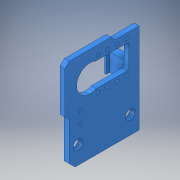
# Autodesk Inventor part: КВ33.044.002 - Деражатель мотора
Saved by Autodesk Inventor 2019 (Build 230136000, 136)
## iProperties
Created: 2019-07-16
Part Number: КВ33.044.002 - Деражатель мотора
Material: Пластик АБС
Document SubType Name: Modeling
Designer: user
Density: 1.06 g/cm^3
Appearance: Голубой
Mass: 13.0069 g
Surface Area: 83.1984 cm^2
Volume: 12.2706 cm^3
Author: user
Autodesk Inventor part; units mm, degrees
ref_plane "YZ Plane" through (0, 0, 0) normal (1, 0, 0) x (0, 1, 0)
ref_plane "XZ Plane" through (0, 0, 0) normal (0, 1, 0) x (-1, 0, 0)
ref_plane "XY Plane" through (0, 0, 0) normal (0, 0, 1) x (1, 0, 0)
sketch "Эскиз1" plane through (0, 0, 0) normal (1, 0, 0) x (0, 1, 0)
  line L0 (-17.5, 21) -> (-21, 17.5)
  line L1 (-21, 17.5) -> (-21, -17.5)
  line L2 (-21, -17.5) -> (-17.5, -21)
  line L3 (-17.5, -21) -> (17.5, -21)
  line L4 (17.5, -21) -> (21, -17.5)
  line L5 (21, -17.5) -> (21, 17.5)
  line L6 (21, 17.5) -> (17.5, 21)
  line L7 (17.5, 21) -> (-17.5, 21)
  circle A0 centre (0, 0) radius 10.75
  circle A1 centre (-15.5, -15.5) radius 1.25
  circle A2 centre (15.5, -15.5) radius 1.25
  circle A3 centre (15.5, 15.5) radius 1.25
  circle A4 centre (-15.5, 15.5) radius 1.25
  line L8 (-21, 17.5) -> (-58, 17.5)
  line L9 (-58, 17.5) -> (-58, -17.5)
  line L10 (-58, -17.5) -> (-21, -17.5)
  line L11 (-21, -17.5) -> (-21, 17.5)
  line L12 (-58, 0) -> (-43, 0)
  line L13 (-43, 0) -> (-43, 10)
  circle A5 centre (-43, 10) radius 4
  circle A6 centre (-43, -33.5) radius 4
  line L14 (-58, -17.5) -> (-17.5, -17.5)
  line L15 (-17.5, -17.5) -> (-17.5, -41)
  line L16 (-17.5, -41) -> (-58, -41)
  line L17 (-58, -41) -> (-58, -17.5)
  dimension "d0" = 37
  dimension "d1" = 15
  dimension "d2" = 10
  dimension "d4" = 8
  dimension "d5" = 8
  dimension "d12" = 21.5
  dimension "d115" = 40.5
  dimension "d116" = 23.5
  dimension "d117" = 7.5
  constraints: 36 end point, 7 centre point, 4 parallel, 3 horizontal, 3 perpendicular, 1 coincident, 1 midpoint
  measures "d0" distance of L10.end L9.end
  measures "d1" distance of L12.start L12.end
  measures "d2" distance of L12.end L13.end
  measures "d4" diameter of A5
  measures "d5" diameter of A6
  measures "d12" diameter of A0
  measures "d115" distance of L15.end L16.end
  measures "d116" distance of L14.end L15.end
  measures "d117" distance from line of L16 A6.centre
extrude "Выдавливание1" add sketch "Эскиз1" along normal blind 4 contours L7 L6 L5 L4 L3 L15 L14 L1 L0 | L1 L10 L9 L8 | L14 L15 L2 | L2 L15 L16 L17 L10 | A0 | A1 | A2 | A3 | A4
chamfer "Фаска1" distance 5 angle 45 1 edges at (2, -58, 17.5)
sketch "Эскиз3" plane through (4, 0, 0) normal (1, 0, 0) x (0, 0, -1)
  line L0 (17.8, -12.6) -> (17.8, -14.9)
  line L1 (17.8, -12.6) -> (19.2, -12.6)
  line L2 (19.2, -14.9) -> (19.2, -12.6)
  line L3 (25.8, -14.9) -> (19.2, -14.9)
  line L4 (25.8, -12.6) -> (25.8, -14.9)
  circle A0 centre (-0.0004, 0.0503) radius 9.15
  circle A1 centre (0, 0) radius 1.5
  circle A2 centre (36, 8) radius 1.3
  circle A3 centre (22.5, 13.5) radius 1.3
  circle A4 centre (30.5, 13.5) radius 1.3
  circle A5 centre (14.5, 13.5) radius 1.3
  circle A6 centre (6.5, 13.5) radius 1.3
  circle A7 centre (36, -8) radius 1.3
  circle A8 centre (22.5, -13.5) radius 1.3
  circle A9 centre (30.5, -13.5) radius 1.3
  circle A10 centre (14.5, -13.5) radius 1.3
  circle A11 centre (6.5, -13.5) radius 1.3
  line L5 (-11.0198, -0.1) -> (-10.4796, -0.1)
  line L6 (-11.0198, -7) -> (-11.0198, -0.1)
  arc A12 (-11.0198, -7) -> (-10.9686, -7.75) centre (-5.5, -7) ccw
  line L7 (-8.5, -7.75) -> (-10.9686, -7.75)
  arc A13 (-6.75, -9.5) -> (-8.5, -7.75) centre (-8.5, -9.5) ccw
  line L8 (-6.75, -10) -> (-6.75, -9.5)
  line L9 (30.8063, -10) -> (-6.75, -10)
  arc A14 (30.8063, -10) -> (31.4945, -9.6078) centre (30.8063, -9.2) ccw
  arc A15 (31.4945, -9.6078) -> (32.1078, -8.9945) centre (33, -10.5) ccw
  arc A16 (32.1078, -8.9945) -> (32.5, -8.3063) centre (31.7, -8.3063) ccw
  line L10 (32.5, 8.3063) -> (32.5, -8.3063)
  arc A17 (32.5, 8.3063) -> (32.1078, 8.9945) centre (31.7, 8.3063) ccw
  arc A18 (31.4945, 9.6078) -> (32.1078, 8.9945) centre (33, 10.5) ccw
  arc A19 (32.1078, 8.9945) -> (31.4945, 9.6078) centre (33, 10.5) ccw
  line L11 (-6.75, -11.3229) -> (-6.75, -10)
  arc A20 (-6.75, -11.3229) -> (-5.5, -11.5) centre (-5.4989, -6.9922) ccw
  line L12 (-5.5, -11.5) -> (2, -11.5)
  line L13 (2, -12.6) -> (2, -11.5)
  line L14 (3.2, -12.6) -> (2, -12.6)
  line L15 (3.2, -14.9) -> (3.2, -12.6)
  line L16 (9.8, -14.9) -> (3.2, -14.9)
  line L17 (9.8, -12.6) -> (9.8, -14.9)
  line L18 (11.2, -12.6) -> (9.8, -12.6)
  line L19 (11.2, -14.9) -> (11.2, -12.6)
  line L20 (17.8, -14.9) -> (11.2, -14.9)
  line L21 (17.8, -12.6) -> (17.8, -14.9)
  line L22 (19.2, -12.6) -> (17.8, -12.6)
  line L23 (19.2, -14.9) -> (19.2, -12.6)
  line L24 (25.8, -14.9) -> (19.2, -14.9)
  line L25 (25.8, -12.6) -> (25.8, -14.9)
  line L26 (27.2, -12.6) -> (25.8, -12.6)
  line L27 (27.2, -14.9) -> (27.2, -12.6)
  line L28 (33.8, -14.9) -> (27.2, -14.9)
  line L29 (33.8, -12.6) -> (33.8, -14.9)
  line L30 (35.0198, -12.6) -> (33.8, -12.6)
  arc A21 (35.0198, -12.6) -> (35.1, -12.5198) centre (34, -11.5) ccw
  line L31 (35.1, -11.3) -> (35.1, -12.5198)
  line L32 (37.4, -11.3) -> (35.1, -11.3)
  line L33 (37.4, -4.7) -> (37.4, -11.3)
  line L34 (35.1, -4.7) -> (37.4, -4.7)
  line L35 (35.1, 4.7) -> (35.1, -4.7)
  line L36 (37.4, 4.7) -> (35.1, 4.7)
  line L37 (37.4, 11.3001) -> (37.4, 4.7)
  line L38 (35.1, 11.3001) -> (37.4, 11.3001)
  line L39 (35.0999, 12.5199) -> (35.1, 11.3001)
  arc A22 (35.0999, 12.5199) -> (35.0197, 12.6001) centre (34, 11.5001) ccw
  line L40 (33.7999, 12.6001) -> (35.0197, 12.6001)
  line L41 (33.7999, 14.9001) -> (33.7999, 12.6001)
  line L42 (27.1999, 14.8999) -> (33.7999, 14.9001)
  line L43 (27.1999, 12.5999) -> (27.1999, 14.8999)
  line L44 (25.7999, 12.5999) -> (27.1999, 12.5999)
  line L45 (25.7999, 14.8999) -> (25.7999, 12.5999)
  line L46 (19.1999, 14.8997) -> (25.7999, 14.8999)
  line L47 (19.1999, 12.5997) -> (19.1999, 14.8997)
  line L48 (17.7999, 12.5997) -> (19.1999, 12.5997)
  line L49 (17.7999, 14.8997) -> (17.7999, 12.5997)
  line L50 (11.1999, 14.8996) -> (17.7999, 14.8997)
  line L51 (11.1999, 12.5996) -> (11.1999, 14.8996)
  line L52 (9.7999, 12.5995) -> (11.1999, 12.5996)
  line L53 (9.7999, 14.8995) -> (9.7999, 12.5995)
  line L54 (3.1999, 14.8994) -> (9.7999, 14.8995)
  line L55 (3.1999, 12.5994) -> (3.1999, 14.8994)
  line L56 (1.9999, 12.5994) -> (3.1999, 12.5994)
  line L57 (2, 11.4994) -> (1.9999, 12.5994)
  line L58 (-5.5, 11.4992) -> (2, 11.4994)
  arc A23 (-5.5, 11.4992) -> (-6.75, 11.3221) centre (-5.4988, 6.9914) ccw
  line L59 (-6.75, 9.9992) -> (-6.75, 11.3221)
  line L60 (-6.75, 9.4992) -> (-6.75, 9.9992)
  arc A24 (-8.5, 7.7491) -> (-6.75, 9.4992) centre (-8.5, 9.4991) ccw
  line L61 (-10.9686, 7.7491) -> (-8.5, 7.7491)
  arc A25 (-10.9686, 7.7491) -> (-11.0197, 6.9991) centre (-5.4999, 6.9992) ccw
  line L62 (-11.0196, 0.0991) -> (-11.0197, 6.9991)
  line L63 (-10.4794, 0.0991) -> (-11.0196, 0.0991)
  arc A26 (32.1078, -8.9945) -> (31.4945, -9.6078) centre (33, -10.5) ccw
  arc A27 (31.4945, 9.6078) -> (30.8063, 10) centre (30.8063, 9.2) ccw
  line L64 (-6.75, 9.9992) -> (30.8063, 10)
  line L65 (-0.0742, 9.2) -> (-0.0742, 9.9993)
  line L66 (-0.0738, -9.0994) -> (-0.0737, -10)
  constraints: 134 end point, 34 point on circle, 28 centre point, 4 point on line, 1 perpendicular
sketch "Эскиз4" plane through (4, 0, 0) normal (1, 0, 0) x (0, 0, -1)
  circle A0 centre (0, 0) radius 11.15
  dimension "d31" = 22.3
  constraints: 1 centre point
  measures "d31" diameter of A0
extrude "Выдавливание4" cut sketch "Эскиз4" against normal blind 10
sketch "Эскиз6" plane through (0, -17.5, -21) normal (0, 0, -1) x (-1, 0, 0)
  line L0 (0, 0) -> (0, 35) projected
  line L1 (0, 35) -> (-4, 35) projected
  line L2 (-4, 0) -> (-4, 35) projected
  line L3 (0, 0) -> (-4, 0) projected
  point P0 (0, 17.5)
extrude "Выдавливание6" add sketch "Эскиз6" along normal blind 20
extrude "Выдавливание7" cut sketch "Эскиз3" against normal blind 15 contours L66 A0 L65 L64 A27 A18 A17 L10 A16 A26 A14 L9 | A3 | A4 | A5 | A6 | A8 | A9 | A10 | A11
sketch "Эскиз14" plane through (0, 0, 0) normal (-1, 0, 0) x (0, 0, 1)
  line L0 (-41, -17.5) -> (-35, -17.5)
  line L1 (-35, -17.5) -> (-35, -7.5)
  line L2 (-35, -7.5) -> (-41, -7.5)
  line L3 (-41, -7.5) -> (-41, -17.5)
  line L4 (-41, -17.5) -> (-35, -17.5)
  line L5 (-35, -17.5) -> (-35, -22.5)
  line L6 (-35, -22.5) -> (-41, -22.5)
  line L7 (-41, -22.5) -> (-41, -17.5)
  point P0 (0, 0)
  dimension "d86" = 6
  dimension "d87" = 10
  dimension "d88" = 6
  dimension "d89" = 5
  constraints: 16 end point, 4 parallel, 2 horizontal, 2 perpendicular
  measures "d86" distance of L2.end L1.end
  measures "d87" distance of L1.end L0.end
  measures "d88" distance of L5.end L6.end
  measures "d89" distance of L4.end L5.end
extrude "Выдавливание15" add sketch "Эскиз14" along normal blind 10
move faces "Перенос2" translate (-6, 0, 0) faces at (-10, -12.5, -39)
sketch "Эскиз15" plane through (0, -22.5, -35) normal (0, 0, 1) x (1, 0, 0)
  line L0 (-16, 0) -> (-16, 15) projected
  line L1 (0, 15) -> (-16, 15) projected
  line L2 (-16, 0) -> (-14.5, 0)
  line L3 (-14.5, 0) -> (-14.5, 15)
  line L4 (-14.5, 15) -> (-16, 15)
  line L5 (-16, 15) -> (-16, 0)
  point P0 (0, 22.5)
  dimension "d95" = 1.5
  constraints: 8 end point, 2 parallel, 1 horizontal, 1 perpendicular, 1 point on line
  measures "d95" distance of L4.end L3.end
extrude "Выдавливание16" add sketch "Эскиз15" along normal blind 3
sketch "Эскиз16" plane through (0, -17.5, -41) normal (0, 0, -1) x (-1, 0, 0)
  line L0 (0, 10) -> (16, 10) projected
  circle A0 centre (7, -2.5) radius 1.6
  line L1 (0, -5) -> (16, -5) projected
  line L2 (16, 10) -> (16, -5) projected
  point P0 (0, 17.5)
  dimension "d99" = 3.2
  dimension "d100" = 2.5
  dimension "d101" = 9
  constraints: 1 centre point
  measures "d99" diameter of A0
  measures "d100" distance from line of L1 A0.centre
  measures "d101" distance from line of L2 A0.centre
extrude "Выдавливание17" cut sketch "Эскиз16" against normal through all
chamfer "Фаска8" distance 3.25 angle 45 1 edges at (-16, -15, -41)
sketch "Эскиз17" plane through (4, 0, 0) normal (1, 0, 0) x (0, 0, -1)
  line L0 (-17.2995, -33.7068) -> (-17.2995, -33.1942)
  line L1 (-17.2995, -33.1942) -> (-15.8655, -33.1025)
  arc A0 (-15.8655, -33.1025) -> (-15.8655, -28.9111) centre (-15.9995, -31.0068) ccw
  line L2 (-15.8655, -28.9111) -> (-17.2995, -28.8194)
  line L3 (-17.2995, -28.8194) -> (-17.2995, -24.531)
  arc A1 (-17.2702, -24.4603) -> (-17.2995, -24.531) centre (-17.1995, -24.531) ccw
  line L4 (-17.2702, -24.4603) -> (-16.946, -24.1361)
  arc A2 (-16.946, -24.1361) -> (-16.7995, -23.7825) centre (-17.2995, -23.7825) ccw
  line L5 (-16.7995, -23.7825) -> (-16.7995, -14.1068)
  line L6 (-7.4495, -14.1068) -> (-7.4495, -17.0325)
  arc A3 (-7.4495, -17.0325) -> (-7.3031, -17.3861) centre (-6.9495, -17.0325) ccw
  line L7 (-7.3031, -17.3861) -> (-6.9788, -17.7103)
  arc A4 (-6.9495, -17.781) -> (-6.9788, -17.7103) centre (-7.0495, -17.781) ccw
  line L8 (-6.9495, -17.781) -> (-6.9495, -20.5325)
  arc A5 (-6.9788, -20.6032) -> (-6.9495, -20.5325) centre (-7.0495, -20.5325) ccw
  line L9 (-6.9788, -20.6032) -> (-7.3031, -20.9275)
  arc A6 (-7.3031, -20.9275) -> (-7.4495, -21.281) centre (-6.9495, -21.281) ccw
  line L10 (-7.4495, -21.281) -> (-7.4495, -26.5325)
  arc A7 (-7.4495, -26.5325) -> (-7.3031, -26.8861) centre (-6.9495, -26.5325) ccw
  line L11 (-7.3031, -26.8861) -> (-6.9788, -27.2103)
  arc A8 (-6.9495, -27.281) -> (-6.9788, -27.2103) centre (-7.0495, -27.281) ccw
  line L12 (-6.9495, -27.281) -> (-6.9495, -30.0325)
  arc A9 (-6.9788, -30.1032) -> (-6.9495, -30.0325) centre (-7.0495, -30.0325) ccw
  line L13 (-6.9788, -30.1032) -> (-7.3031, -30.4275)
  arc A10 (-7.3031, -30.4275) -> (-7.4495, -30.781) centre (-6.9495, -30.781) ccw
  line L14 (-7.4495, -30.781) -> (-7.4495, -33.7068)
  arc A11 (-7.5495, -33.8068) -> (-7.4495, -33.7068) centre (-7.5495, -33.7068) ccw
  line L15 (-7.5495, -33.8068) -> (-17.1995, -33.8068)
  arc A12 (-17.2995, -33.7068) -> (-17.1995, -33.8068) centre (-17.1995, -33.7068) ccw
  circle A13 centre (-8.1696, -28.6568) radius 1.25
  circle A14 centre (-8.1696, -19.1568) radius 1.25
  line L16 (-7.4495, -14.1068) -> (-16.7995, -14.1068)
  point P0 (0, 0)
  point P1 (-8.1696, -28.6568)
  constraints: 34 end point, 26 point on circle, 15 centre point, 1 horizontal
extrude "Выдавливание18" cut sketch "Эскиз17" against normal through all contours A13 L12 | L12 A13 | A14 L8 | L8 A14
sketch "Эскиз18" plane through (4, 0, 0) normal (1, 0, 0) x (0, 0, -1)
  circle A0 centre (-8.1696, -19.1568) radius 1.25 projected
  circle A1 centre (-8.1696, -28.6568) radius 1.25 projected
  line L0 (30.8063, -10) -> (4.9318, -10) projected
  arc A2 (4.9329, 9.9994) -> (4.9318, -10) centre (0, 0) ccw projected
  line L1 (4.9329, 9.9994) -> (30.8063, 10) projected
  arc A3 (31.4945, 9.6078) -> (30.8063, 10) centre (30.8063, 9.2) ccw projected
  arc A4 (31.4945, 9.6078) -> (32.1078, 8.9945) centre (33, 10.5) ccw projected
  arc A5 (32.5, 8.3063) -> (32.1078, 8.9945) centre (31.7, 8.3063) ccw projected
  line L2 (32.5, 8.3063) -> (32.5, -8.3063) projected
  arc A6 (32.1078, -8.9945) -> (32.5, -8.3063) centre (31.7, -8.3063) ccw projected
  arc A7 (32.1078, -8.9945) -> (31.4945, -9.6078) centre (33, -10.5) ccw projected
  arc A8 (30.8063, -10) -> (31.4945, -9.6078) centre (30.8063, -9.2) ccw projected
  circle A9 centre (14.5, -13.5) radius 1.3 projected
  circle A10 centre (22.5, -13.5) radius 1.3 projected
  circle A11 centre (14.5, 13.5) radius 1.3 projected
  circle A12 centre (22.5, 13.5) radius 1.3 projected
  circle A13 centre (30.5, 13.5) radius 1.3 projected
  circle A14 centre (6.5, 13.5) radius 1.3 projected
  circle A15 centre (30.5, -13.5) radius 1.3 projected
  circle A16 centre (6.5, -13.5) radius 1.3 projected
  line L3 (21, 17.5) -> (41, 17.5) projected
  line L4 (21, 17.5) -> (17.5, 21) projected
  line L5 (17.5, 21) -> (-17.5, 21) projected
  line L6 (-17.5, 21) -> (-21, 17.5) projected
  line L7 (-21, 17.5) -> (-21, -17.5) projected
  line L8 (-21, -17.5) -> (-17.5, -21) projected
  line L9 (-17.5, -21) -> (-17.5, -53) projected
  line L10 (-12.5, -58) -> (-17.5, -53) projected
  line L11 (-12.5, -58) -> (41, -58) projected
  circle A17 centre (-10, -43) radius 4 projected
  line L12 (41, -58) -> (41, 17.5) projected
